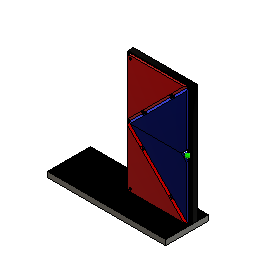
Evolution_door (Autodesk Fusion 360 design; units mm, degrees)
Autodesk Fusion 360 part; units mm, degrees
sketch "Frame" plane through (0, 0, 0) normal (0, 0, 1) x (1, 0, 0) in component "Door frame"
  line L0 (0, 0) -> (50, 0)
  line L1 (50, 0) -> (50, 100)
  line L2 (50, 100) -> (0, 100)
  line L3 (0, 100) -> (0, 0)
  line L4 (-5, -5) -> (55, -5)
  line L5 (55, -5) -> (55, 105)
  line L6 (55, 105) -> (-5, 105)
  line L7 (-5, 105) -> (-5, -5)
  dimension "d1" = 5
  constraint horizontal L0
  constraint vertical L1
  constraint horizontal L2
  constraint vertical L3
  constraint coincident L0.start L3.end
extrude "Extrude1" add sketch "Frame" against normal blind 5 makes body 1 in component "Door frame"
sketch "Body" plane through (0, 0, 0) normal (0, 0, 1) x (1, 0, 0) in component "Triangle1"
  line L0 (0, 0) -> (0, 100) construction
  line L1 (0, 100) -> (50, 100) construction
  line L2 (50, 100) -> (50, 0)
  line L3 (50, 0) -> (0, 0)
  line L4 (-5, 105) -> (-5, -5)
  line L5 (-5, -5) -> (55, -5)
  line L6 (55, -5) -> (55, 105)
  line L7 (55, 105) -> (-5, 105)
  line L8 (0, 100) -> (-5, 105) construction
  line L9 (50, 100) -> (55, 105) construction
  line L10 (-5, 50) -> (55, 50) construction
  line L11 (-2.5, 105) -> (-2.5, 50) construction
  line L12 (52.5, 105) -> (52.5, 50) construction
  line L13 (52.5, 105) -> (-2.5, 105) construction
  line L14 (52.5, 105) -> (-2.5, 50) construction
  line L15 (50, 100) -> (50, 105) construction
  line L16 (-2.5, 50) -> (-2.5, 52.5) construction
  line L17 (50, 105) -> (-2.5, 52.5)
  line L18 (-2.5, 52.5) -> (-2.5, 105)
  line L19 (-2.5, 105) -> (2.5, 105) construction
  line L20 (2.5, 105) -> (2.5, 100) construction
  line L21 (2.5, 100) -> (-2.5, 100) construction
  line L22 (-2.5, 100) -> (-2.5, 105) construction
  circle A0 centre (0, 102.5) radius 1.1
  line L23 (23.75, 78.75) -> (50, 105)
  line L24 (36.875, 91.875) -> (38.125, 90.625)
  line L25 (23.75, 78.75) -> (-2.5, 52.5)
  line L26 (10.625, 65.625) -> (11.875, 64.375)
  line L27 (10.625, 65.625) -> (11.3321, 66.3321)
  line L28 (11.3321, 66.3321) -> (12.5821, 65.0821)
  line L29 (11.875, 64.375) -> (12.5821, 65.0821)
  line L30 (36.875, 91.875) -> (37.5821, 92.5821)
  line L31 (37.5821, 92.5821) -> (38.8321, 91.3321)
  line L32 (38.125, 90.625) -> (38.8321, 91.3321)
  line L33 (11.875, 64.375) -> (12.5821, 63.6679)
  line L34 (12.5821, 65.0821) -> (13.2892, 64.375)
  line L35 (12.5821, 63.6679) -> (13.2892, 64.375)
  line L36 (11.875, 64.375) -> (11.1679, 65.0821)
  line L37 (11.1679, 65.0821) -> (11.875, 65.7892)
  line L38 (11.5214, 64.7286) -> (12.2286, 65.4357)
  line L39 (12.2286, 64.0214) -> (12.9357, 64.7286)
  line L40 (38.125, 90.625) -> (37.4179, 91.3321)
  line L41 (37.4179, 91.3321) -> (38.125, 92.0392)
  line L42 (37.7714, 90.9786) -> (38.4786, 91.6857)
  line L43 (38.125, 90.625) -> (38.8321, 89.9179)
  line L44 (38.8321, 91.3321) -> (39.5392, 90.625)
  line L45 (38.8321, 89.9179) -> (39.5392, 90.625)
  line L46 (38.4786, 90.2714) -> (39.1857, 90.9786)
  line L47 (-2.5, 52.5) -> (-2.5, 50.5)
  line L48 (10.625, 65.625) -> (9.2108, 64.2108)
  line L49 (36.875, 91.875) -> (35.4608, 90.4608)
  line L50 (-2.5, 50.5) -> (-2.5, 50)
  line L51 (10.8143, 63.3143) -> (-2.5, 50)
  line L52 (52.5, 105) -> (38.8321, 91.3321)
  line L53 (37.0643, 89.5643) -> (12.5821, 65.0821)
  line L54 (9.2108, 64.2108) -> (10.4608, 62.9608)
  line L55 (35.4608, 90.4608) -> (36.7101, 89.2101)
  line L56 (52.5, 105) -> (-2.5, 105)
  dimension "d4" = 2.5
  dimension "d5" = 5
  dimension "d6" = 5
  dimension "d7" = 2.2
  dimension "d43" = 1
  dimension "d44" = 1
  dimension "d45" = 1
  dimension "d46" = 1
  dimension "d47" = 1
  dimension "d48" = 1
  dimension "d49" = 1
  dimension "d50" = 1
  dimension "d196" = 2
  dimension "d198" = 2
  constraint coincident L0.end L1.start
  constraint coincident L4.start L7.end
  constraint coincident L1.end L2.start
  constraint coincident L6.end L7.start
  constraint midpoint L4 L10.start
  constraint midpoint L6 L10.end
  constraint coincident L7 L11.start
  constraint coincident L10 L11.end
  constraint perpendicular L10 L11
  constraint coincident L7 L12.start
  constraint coincident L13 L15.end
  constraint perpendicular L10 L16
  constraint horizontal L19
  constraint vertical L20
  constraint horizontal L21
  constraint vertical L22
  constraint midpoint L17 L23.start
  constraint midpoint L23 L24.start
  constraint coincident L14 L24.end
  constraint perpendicular L14 L24
  constraint midpoint L25 L26.start
  constraint coincident L14 L26.end
  constraint perpendicular L14 L26
  constraint perpendicular L26 L27
  constraint coincident L14 L28.end
  constraint perpendicular L14 L28
  constraint perpendicular L24 L30
  constraint coincident L14 L31.end
  constraint perpendicular L14 L31
  constraint perpendicular L29 L33
  constraint perpendicular L14 L34
  constraint perpendicular L29 L36
  constraint coincident L28 L37.end
  constraint perpendicular L28 L37
  constraint midpoint L36 L38.start
  constraint coincident L28 L38.end
  constraint perpendicular L28 L38
  constraint midpoint L33 L39.start
  constraint midpoint L34 L39.end
  constraint perpendicular L32 L40
  constraint coincident L31 L41.end
  constraint perpendicular L31 L41
  constraint midpoint L40 L42.start
  constraint perpendicular L24 L42
  constraint perpendicular L32 L43
  constraint perpendicular L32 L44
  constraint midpoint L43 L46.start
  constraint midpoint L44 L46.end
  constraint coincident L11 L47.end
  constraint parallel L11 L47
  constraint perpendicular L26 L48
  constraint perpendicular L24 L49
  constraint parallel L11 L50
  constraint coincident L14 L51.start
  constraint coincident L14 L53.start
  constraint coincident L51 L54.end
  constraint coincident L14 L54.end
  constraint coincident L53 L55.end
  measures "d4" distance of L11.end L16.end
  measures "d5" distance of L11.start L19.end
  measures "d6" distance of L11.start L21.end
  measures "d7" diameter of A0
  measures "d43" distance of L26.start L27.end
  measures "d44" distance of L24.start L30.end
  measures "d45" distance of L26.end L33.end
  measures "d46" distance of L28.end L34.end
  measures "d47" distance of L26.end L36.end
  measures "d48" distance of L24.end L40.end
  measures "d49" distance of L24.end L43.end
  measures "d50" distance of L31.end L44.end
  measures "d196" distance of L26.start L48.end
  measures "d198" distance of L24.start L49.end
extrude "Extrude1'" add sketch "Body" along normal blind 3 and the other way blind -1 separate body contours L7 L17 L18 L23 L25 L27 L30 L48 L49 L56 makes body 2 in component "Triangle1"
sketch "Triangle1 holder" plane through (0, 0, 0) normal (0, 0, 1) x (1, 0, 0) in component "Door frame"
  line L0 (0, 0) -> (0, 100)
  line L1 (0, 100) -> (50, 100)
  line L2 (50, 100) -> (50, 0)
  line L3 (50, 0) -> (0, 0)
  line L4 (-5, 105) -> (-5, -5)
  line L5 (-5, -5) -> (55, -5)
  line L6 (55, -5) -> (55, 105)
  line L7 (55, 105) -> (-5, 105)
  circle A0 centre (0, 102.5) radius 1
  circle A1 centre (0, 102.5) radius 1.5
  dimension "d12" = 2
  dimension "d13" = 3
  constraint concentric A0 A1
  measures "d12" diameter of A0
  measures "d13" diameter of A1
extrude "Extrude2" add sketch "Triangle1 holder" along normal blind 0.8 contours A1 bodies 1 in component "Door frame"
extrude "Extrude3" add 1 faces at (0.2444, 102.8261, 0) along direction (0, 0, 1) blind 3 on bodies 1 bodies 1 in component "Door frame"
sketch "Body (2)" plane through (0, 0, 0) normal (0, 0, 1) x (1, 0, 0) in component "Triangle4"
  line L0 (-5, 105) -> (-5, -5)
  line L1 (-5, -5) -> (55, -5)
  line L2 (55, -5) -> (55, 105)
  line L3 (55, 105) -> (-5, 105)
  line L4 (0, 0) -> (0, 100) construction
  line L5 (0, 100) -> (50, 100)
  line L6 (50, 100) -> (50, 0)
  line L7 (50, 0) -> (0, 0) construction
  circle A0 centre (0, 102.5) radius 1.5
  line L8 (-5, -5) -> (0, 0) construction
  line L9 (50, 0) -> (55, -5) construction
  line L10 (-5, 50) -> (55, 50) construction
  line L11 (52.5, -2.5) -> (52.5, -5) construction
  line L12 (-2.5, -2.5) -> (-2.5, -5) construction
  line L13 (-2.5, -5) -> (-2.5, 50) construction
  line L14 (52.5, -5) -> (52.5, 50) construction
  line L15 (50, 0) -> (50, -5) construction
  line L16 (-2.5, -5) -> (50, -5) construction
  line L17 (-2.5, -5) -> (-2.5, 47.5)
  line L18 (-2.5, 47.5) -> (50, -5)
  circle A1 centre (0, -2.5) radius 1.1
  line L19 (-2.5, 50) -> (52.5, -5) construction
  line L20 (23.75, 21.25) -> (50, -5)
  line L21 (36.875, 8.125) -> (38.125, 9.375)
  line L22 (-2.5, 47.5) -> (23.75, 21.25)
  line L23 (10.625, 34.375) -> (11.875, 35.625)
  line L24 (10.625, 34.375) -> (11.3321, 33.6679)
  line L25 (11.3321, 33.6679) -> (12.5821, 34.9179)
  line L26 (11.875, 35.625) -> (12.5821, 34.9179)
  line L27 (11.875, 35.625) -> (11.5214, 35.2714)
  line L28 (11.5214, 35.2714) -> (12.2286, 34.5643)
  line L29 (11.875, 35.625) -> (12.5821, 36.3321)
  line L30 (12.5821, 34.9179) -> (13.2892, 35.625)
  line L31 (12.5821, 36.3321) -> (13.2892, 35.625)
  line L32 (12.2286, 35.9786) -> (12.9357, 35.2714)
  line L33 (36.875, 8.125) -> (37.5821, 7.4179)
  line L34 (37.5821, 7.4179) -> (38.8321, 8.6679)
  line L35 (38.125, 9.375) -> (37.7714, 9.0214)
  line L36 (37.7714, 9.0214) -> (38.4786, 8.3143)
  line L37 (38.125, 9.375) -> (38.8321, 10.0821)
  line L38 (38.8321, 10.0821) -> (39.5392, 9.375)
  line L39 (39.5392, 9.375) -> (38.8321, 8.6679)
  line L40 (38.4786, 9.7286) -> (39.1857, 9.0214)
  line L41 (-2.5, 47.5) -> (-2.5, 50)
  line L42 (10.625, 34.375) -> (9.2108, 35.7892)
  line L43 (9.2108, 35.7892) -> (10.4608, 37.0392)
  line L44 (36.875, 8.125) -> (35.4608, 9.5392)
  line L45 (35.4608, 9.5392) -> (36.7108, 10.7892)
  line L46 (-2.5, 50) -> (10.4608, 37.0392)
  line L47 (12.5821, 34.9179) -> (36.7108, 10.7892)
  line L48 (38.8321, 8.6679) -> (52.5, -5)
  dimension "d25" = 2.2
  dimension "d61" = 1
  dimension "d62" = 0.5
  dimension "d63" = 1
  dimension "d64" = 1
  dimension "d65" = 1
  dimension "d66" = 0.5
  dimension "d67" = 1
  dimension "d206" = 2
  dimension "d207" = 2
  constraint coincident L0.end L1.start
  constraint coincident L4.start L7.end
  constraint coincident L6.end L7.start
  constraint coincident L1.end L2.start
  constraint midpoint L0 L10.start
  constraint perpendicular L0 L10
  constraint midpoint L9 L11.start
  constraint coincident L1 L11.end
  constraint perpendicular L1 L11
  constraint midpoint L8 L12.start
  constraint coincident L1 L12.end
  constraint perpendicular L1 L12
  constraint coincident L10 L13.end
  constraint perpendicular L10 L13
  constraint perpendicular L1 L14
  constraint coincident L13 L17.end
  constraint midpoint L18 L20.start
  constraint midpoint L20 L21.start
  constraint coincident L19 L21.end
  constraint perpendicular L19 L21
  constraint midpoint L22 L23.start
  constraint coincident L19 L23.end
  constraint perpendicular L19 L23
  constraint perpendicular L23 L24
  constraint coincident L19 L25.end
  constraint perpendicular L19 L25
  constraint perpendicular L26 L27
  constraint coincident L25 L28.end
  constraint perpendicular L25 L28
  constraint perpendicular L19 L29
  constraint perpendicular L19 L30
  constraint midpoint L29 L32.start
  constraint midpoint L30 L32.end
  constraint perpendicular L21 L33
  constraint coincident L19 L34.end
  constraint perpendicular L19 L34
  constraint perpendicular L19 L35
  constraint coincident L34 L36.end
  constraint perpendicular L34 L36
  constraint perpendicular L19 L37
  constraint perpendicular L37 L38
  constraint midpoint L37 L40.start
  constraint midpoint L39 L40.end
  constraint perpendicular L23 L42
  constraint coincident L19 L43.end
  constraint perpendicular L19 L43
  constraint perpendicular L43 L44
  constraint coincident L19 L45.end
  constraint perpendicular L19 L45
  measures "d25" diameter of A1
  measures "d61" distance of L23.start L24.end
  measures "d62" distance of L23.end L27.end
  measures "d63" distance of L23.end L29.end
  measures "d64" distance of L25.end L30.end
  measures "d65" distance of L21.start L33.end
  measures "d66" distance of L21.end L35.end
  measures "d67" distance of L21.end L37.end
  measures "d206" distance of L23.start L42.end
  measures "d207" distance of L21.start L44.end
extrude "Extrude1''" add sketch "Body (2)" along normal blind 3 and the other way blind -1 separate body contours L1 L17 L18 L20 L22 L24 L33 L42 L44 makes body 3 in component "Triangle4"
sketch "Sketch3" plane through (0, 0, 0) normal (0, 0, 1) x (1, 0, 0) in component "Door frame"
  line L0 (-5, 105) -> (-5, -5)
  line L1 (-5, -5) -> (55, -5)
  line L2 (55, -5) -> (55, 105)
  line L3 (55, 105) -> (-5, 105)
  line L4 (0, 0) -> (0, 100)
  line L5 (0, 100) -> (50, 100)
  line L6 (50, 100) -> (50, 0)
  line L7 (50, 0) -> (0, 0)
  circle A0 centre (0, 102.5) radius 1.5
  circle A1 centre (0, -2.5) radius 1
  circle A2 centre (0, -2.5) radius 1.5
  dimension "d30" = 2
  dimension "d31" = 3
  constraint concentric A1 A2
  measures "d30" diameter of A1
  measures "d31" diameter of A2
extrude "Extrude4" add sketch "Sketch3" along normal blind 0.8 contours A2 bodies 1 in component "Door frame"
extrude "Extrude5" add 1 faces at (0.5696, -2.7503, 0) along direction (0, 0, 1) blind 3 on bodies 1 bodies 1 in component "Door frame"
extrude "Extrude2'" add sketch "Body" along normal blind 3 and the other way blind -1 contours L17 L23 L24 L30 L31 L41 | L24 L31 L32 L40 L42 | L32 L43 L44 L46 | L24 L31 L40 L41 L42 | L17 L25 L26 L27 L28 L37 | L43 L44 L45 L46 | L26 L28 L36 L37 L38 | L26 L28 L29 L36 L38 | L29 L33 L34 L39 | L33 L34 L35 L39 bodies 2 in component "Triangle1"
extrude "Extrude3'" cut sketch "Body" along normal blind 2.5 and the other way blind -1.5 contours L24 L31 L32 L40 L42 | L32 L43 L44 L46 | L26 L28 L29 L36 L38 | L29 L33 L34 L39 bodies 2 in component "Triangle1"
fillet "Fillet2" radius 1 4 edges at (12.9357, 64.0214, 1) (12.9357, 64.0214, 3) (39.1857, 90.2714, 1) (39.1857, 90.2714, 3) on bodies 2 in component "Triangle1"
extrude "Extrude2''" add sketch "Body (2)" along normal blind 3 and the other way blind -1 contours L18 L20 L21 L33 L34 L36 | L21 L34 L35 L36 L37 L39 L40 | L18 L22 L23 L24 L25 L28 | L37 L38 L39 L40 | L23 L25 L26 L27 L28 | L26 L29 L30 L32 | L29 L30 L31 L32 bodies 3 in component "Triangle4"
extrude "Extrude3''" cut sketch "Body (2)" along normal blind 2.5 and the other way blind -1.5 contours L21 L34 L35 L36 L37 L39 L40 | L23 L25 L26 L27 L28 | L26 L29 L30 L32 bodies 3 in component "Triangle4"
fillet "Fillet1" radius 1 4 edges at (12.9357, 35.9786, 3) (12.9357, 35.9786, 1) (39.1857, 9.7286, 3) (39.1857, 9.7286, 1) on bodies 3 in component "Triangle4"
sketch "Body (3)" plane through (0, 0, 0) normal (0, 0, 1) x (1, 0, 0) in component "Triangle2"
  circle A0 centre (0, 102.5) radius 1.5
  line L0 (0, 0) -> (0, 100)
  line L1 (0, 100) -> (50, 100) construction
  line L2 (50, 100) -> (50, 0) construction
  line L3 (50, 0) -> (0, 0)
  line L4 (-5, 105) -> (-5, -5)
  line L5 (-5, -5) -> (55, -5)
  line L6 (55, -5) -> (55, 105)
  line L7 (55, 105) -> (-5, 105)
  circle A1 centre (0, -2.5) radius 1.5
  line L8 (-5, 105) -> (0, 100) construction
  line L9 (50, 100) -> (55, 105) construction
  line L10 (52.5, 102.5) -> (52.5, 105) construction
  line L11 (-2.5, 105) -> (-2.5, 50) construction
  line L12 (52.5, 105) -> (52.5, 50.7071) construction
  line L13 (-2.5, 50) -> (-2.5, 105) construction
  line L14 (-2.5, 50) -> (52.5, 105) construction
  line L15 (0, 50) -> (0, 52.5) construction
  line L16 (0, 50) -> (52.5, 102.5) construction
  line L17 (0, 52.5) -> (2.5, 52.5) construction
  line L18 (50, 100) -> (50, 102.5) construction
  line L19 (50, 100) -> (2.5, 52.5)
  line L20 (2.5, 52.5) -> (50, 52.5)
  line L21 (50, 52.5) -> (50, 100)
  line L22 (26.25, 76.25) -> (0, 50) construction
  line L23 (13.125, 63.125) -> (11.875, 64.375)
  line L24 (13.125, 63.125) -> (12.4179, 62.4179)
  line L25 (12.4179, 62.4179) -> (11.1679, 63.6679)
  line L26 (11.1679, 63.6679) -> (10.8143, 64.0214)
  line L27 (11.875, 64.375) -> (11.5214, 64.7286)
  line L28 (11.5214, 64.7286) -> (12.2293, 65.4364)
  line L29 (12.2293, 65.4364) -> (12.9371, 64.7286)
  line L30 (12.9371, 64.7286) -> (12.2293, 64.0207)
  line L31 (26.25, 76.25) -> (52.5, 102.5) construction
  line L32 (39.375, 89.375) -> (38.125, 90.625)
  line L33 (39.375, 89.375) -> (38.6679, 88.6679)
  line L34 (38.6679, 88.6679) -> (37.4179, 89.9179)
  line L35 (37.4179, 89.9179) -> (37.0643, 90.2714)
  line L36 (37.7714, 90.9786) -> (38.125, 90.625)
  line L37 (37.7714, 90.9786) -> (38.4786, 91.6857)
  line L38 (38.4786, 91.6857) -> (39.1857, 90.9786)
  line L39 (39.1857, 90.9786) -> (38.4786, 90.2714)
  line L40 (37.0643, 90.2714) -> (36.7108, 90.625)
  line L41 (37.7714, 90.9786) -> (37.4179, 91.3321)
  line L42 (36.7108, 90.625) -> (37.4179, 91.3321)
  line L43 (10.8143, 64.0214) -> (10.4608, 64.375)
  line L44 (11.5214, 64.7286) -> (11.1679, 65.0821)
  line L45 (11.1679, 65.0821) -> (10.4608, 64.375)
  line L46 (50, 52.5) -> (52.5, 50) construction
  line L47 (13.125, 63.125) -> (14.5392, 64.5392)
  line L48 (14.5392, 64.5392) -> (13.2892, 65.7892)
  line L49 (39.375, 89.375) -> (40.7892, 90.7892)
  line L50 (40.7892, 90.7892) -> (39.5392, 92.0392)
  line L51 (50, 102.5) -> (39.5392, 92.0392)
  line L52 (37.4179, 89.9179) -> (13.2892, 65.7892)
  line L53 (-2.5, 50) -> (11.1679, 63.6679)
  line L54 (50, 102.5) -> (52.5, 105)
  line L55 (52.5, 105) -> (52.5, 50.7071)
  line L56 (2.5, 52.5) -> (0, 50)
  line L57 (50, 100) -> (52.5, 102.5)
  line L58 (50, 52.5) -> (52.5, 55)
  line L59 (50, 52.5) -> (53.5355, 52.5) construction
  line L60 (50, 52.5) -> (47.5, 50)
  line L61 (50.3536, 52.8536) -> (52.8539, 50.3532)
  line L62 (52.8539, 50.3532) -> (52.1468, 49.6461)
  line L63 (52.1468, 49.6461) -> (49.6464, 52.1464)
  line L64 (51.7929, 50) -> (50, 50)
  line L65 (47.5, 50) -> (-2.5, 50)
  line L66 (50, 50) -> (47.5, 50)
  line L67 (52.5, 50.7071) -> (52.5, 50) construction
  line L68 (-5, 50) -> (51.7929, 50) construction
  line L69 (52.5, 50) -> (55, 50) construction
  line L70 (51.7929, 50) -> (52.5, 50) construction
  line L71 (52.5, 50) -> (51.7929, 50) construction
  line L72 (52.5, 50.7071) -> (52.5, 50) construction
  dimension "d77" = 1
  dimension "d78" = 0.5
  dimension "d79" = 0.5
  dimension "d80" = 1
  dimension "d81" = 0.5
  dimension "d82" = 1
  dimension "d83" = 1
  dimension "d84" = 1
  dimension "d94" = 0.5
  dimension "d95" = 0.5
  dimension "d96" = 0.5
  dimension "d97" = 0.5
  dimension "d214" = 2
  dimension "d215" = 2
  dimension "d252" = 45
  dimension "d254" = 3.536
  dimension "d255" = 1
  constraint midpoint L4 L68.start
  constraint midpoint L6 L69.end
  constraint coincident L4.start L7.end
  constraint coincident L0.end L1.start
  constraint coincident L1.end L2.start
  constraint coincident L6.end L7.start
  constraint midpoint L9 L10.start
  constraint coincident L7 L10.end
  constraint perpendicular L7 L10
  constraint coincident L7 L11.start
  constraint coincident L11.end L68
  constraint perpendicular L11 L68
  constraint coincident L46.end L68
  constraint perpendicular L12 L68
  constraint midpoint L0 L15.start
  constraint coincident L0 L15.end
  constraint coincident L14 L15.end
  constraint coincident L16 L17.end
  constraint perpendicular L15 L17
  constraint coincident L14 L18.end
  constraint perpendicular L1 L18
  constraint coincident L2 L20.end
  constraint perpendicular L2 L20
  constraint midpoint L19 L22.start
  constraint midpoint L22 L23.start
  constraint coincident L14 L23.end
  constraint perpendicular L14 L23
  constraint perpendicular L23 L24
  constraint coincident L14 L25.end
  constraint perpendicular L14 L25
  constraint perpendicular L14 L26
  constraint perpendicular L14 L27
  constraint perpendicular L27 L28
  constraint perpendicular L28 L29
  constraint coincident L23 L30.end
  constraint perpendicular L23 L30
  constraint midpoint L31 L32.start
  constraint coincident L14 L32.end
  constraint perpendicular L14 L32
  constraint perpendicular L32 L33
  constraint coincident L14 L34.end
  constraint perpendicular L14 L34
  constraint perpendicular L14 L35
  constraint perpendicular L36 L37
  constraint perpendicular L37 L38
  constraint coincident L32 L39.end
  constraint perpendicular L32 L39
  constraint parallel L35 L40
  constraint perpendicular L37 L41
  constraint perpendicular L41 L42
  constraint parallel L26 L43
  constraint perpendicular L28 L44
  constraint perpendicular L23 L47
  constraint coincident L14 L48.end
  constraint perpendicular L14 L48
  constraint perpendicular L32 L49
  constraint coincident L14 L50.end
  constraint perpendicular L14 L50
  constraint coincident L15.end L53
  constraint horizontal L59
  constraint coincident L55 L58.end
  constraint coincident L60.end L64
  constraint parallel L58 L60
  constraint perpendicular L46 L62
  constraint coincident L60 L63.end
  constraint perpendicular L60 L63
  constraint coincident L2 L64.end
  constraint coincident L61 L12.end
  constraint perpendicular L67 L68
  constraint coincident L63 L64.start
  constraint coincident L60.end L71
  constraint coincident L58.end L72
  measures "d77" distance of L23.start L24.end
  measures "d78" distance of L25.end L26.end
  measures "d79" distance of L23.end L27.end
  measures "d80" distance of L32.start L33.end
  measures "d81" distance of L34.end L35.end
  measures "d82" distance of L35.end L36.start
  measures "d83" distance of L36.start L37.end
  measures "d84" distance of L37.end L38.end
  measures "d94" distance of L35.end L40.end
  measures "d95" distance of L36.start L41.end
  measures "d96" distance of L26.end L43.end
  measures "d97" distance of L27.end L44.end
  measures "d214" distance of L23.start L47.end
  measures "d215" distance of L32.start L49.end
  measures "d252" angle of L58 L59
  measures "d254" distance of L61.start L61.end
  measures "d255" distance of L61.end L62.end
extrude "Extrude1'''" add sketch "Body (3)" along normal blind 3 and the other way blind -1 separate body contours L20 L56 L60 L65 | L19 L20 L21 L24 L33 L47 L49 | L19 L23 L24 L25 L26 L27 L43 L44 L45 | L21 L55 L57 L58 | L19 L32 L33 L34 L35 L36 L40 L41 L42 makes body 4 in component "Triangle2"
extrude "Extrude2'''" add sketch "Body (3)" along normal blind 2.5 and the other way blind -1.5 contours L23 L27 L28 L29 L30 | L32 L36 L37 L38 L39 bodies 4 in component "Triangle2"
fillet "Fillet1'" radius 0.5 8 edges at (11.8754, 65.0825, 2.5) (12.5832, 64.3746, 2.5) (11.8754, 65.0825, 1.5) (12.5832, 64.3746, 1.5) (38.125, 91.3321, 1.5) (38.8321, 90.625, 1.5) (38.125, 91.3321, 2.5) (38.8321, 90.625, 2.5) on bodies 4 in component "Triangle2"
fillet "Fillet2'" radius 1 4 edges at (37.0643, 90.9786, 3) (37.0643, 90.9786, 1) (10.8143, 64.7286, 1) (10.8143, 64.7286, 3) on bodies 4 in component "Triangle2"
sketch "Body (4)" plane through (0, 0, 0) normal (0, 0, 1) x (1, 0, 0) in component "Triangle3"
  circle A0 centre (0, 102.5) radius 1.5
  line L0 (0, 0) -> (0, 100) construction
  line L1 (0, 100) -> (50, 100)
  line L2 (50, 100) -> (50, 0) construction
  line L3 (50, 0) -> (0, 0) construction
  line L4 (-5, 105) -> (-5, -5)
  line L5 (-5, -5) -> (55, -5)
  line L6 (55, -5) -> (55, 105)
  line L7 (55, 105) -> (-5, 105)
  circle A1 centre (0, -2.5) radius 1.5
  line L8 (-5, 50) -> (55, 50) construction
  line L9 (-5, -5) -> (0, 0) construction
  line L10 (55, -5) -> (50, 0) construction
  line L11 (52.5, -2.5) -> (52.5, -5) construction
  line L12 (-2.5, -2.5) -> (-2.5, -5) construction
  line L13 (-2.5, -5) -> (-2.5, 50) construction
  line L14 (52.5, -5) -> (52.5, 50) construction
  line L15 (-2.5, 50) -> (52.5, -5) construction
  line L16 (-2.5, 50) -> (0, 50) construction
  line L17 (0, 47.5) -> (2.5, 47.5) construction
  line L18 (50, 0) -> (50, -2.5) construction
  line L19 (2.5, 47.5) -> (50, 0)
  line L20 (2.5, 47.5) -> (50, 47.5)
  line L21 (50, 47.5) -> (50, 0)
  line L22 (0, 50) -> (52.5, -2.5) construction
  line L23 (26.25, 23.75) -> (0, 50) construction
  line L24 (13.125, 36.875) -> (11.875, 35.625)
  line L25 (11.875, 35.625) -> (11.1679, 34.9179)
  line L26 (13.125, 36.875) -> (12.4179, 37.5821)
  line L27 (12.4179, 37.5821) -> (11.1679, 36.3321)
  line L28 (11.1679, 36.3321) -> (10.4608, 35.625)
  line L29 (11.1679, 34.9179) -> (10.4608, 35.625)
  line L30 (11.5214, 35.2714) -> (10.8143, 35.9786)
  line L31 (11.875, 35.625) -> (12.2286, 35.9786)
  line L32 (12.2286, 35.9786) -> (11.5214, 36.6857)
  line L33 (26.25, 23.75) -> (52.5, -2.5) construction
  line L34 (39.375, 10.625) -> (38.125, 9.375)
  line L35 (39.375, 10.625) -> (38.6679, 11.3321)
  line L36 (38.6679, 11.3321) -> (37.4179, 10.0821)
  line L37 (37.4179, 10.0821) -> (36.7108, 9.375)
  line L38 (38.125, 9.375) -> (37.4179, 8.6679)
  line L39 (37.4179, 8.6679) -> (36.7108, 9.375)
  line L40 (37.7714, 9.0214) -> (37.0643, 9.7286)
  line L41 (38.125, 9.375) -> (38.4786, 9.7286)
  line L42 (38.4786, 9.7286) -> (37.7714, 10.4357)
  line L43 (11.5214, 35.2714) -> (12.2286, 34.5643)
  line L44 (12.2286, 34.5643) -> (12.9357, 35.2714)
  line L45 (12.9357, 35.2714) -> (12.2286, 35.9786)
  line L46 (37.7714, 9.0214) -> (38.4786, 8.3143)
  line L47 (38.4786, 8.3143) -> (39.1857, 9.0214)
  line L48 (39.1857, 9.0214) -> (38.4786, 9.7286)
  line L49 (50, 47.5) -> (52.5, 50) construction
  line L50 (51.25, 48.75) -> (51.6036, 48.3964) construction
  line L51 (13.125, 36.875) -> (14.5392, 35.4608)
  line L52 (14.5392, 35.4608) -> (13.2892, 34.2108)
  line L53 (13.2892, 34.2108) -> (37.4179, 10.0821)
  line L54 (39.375, 10.625) -> (40.7892, 9.2108)
  line L55 (40.7892, 9.2108) -> (39.5392, 7.9608)
  line L56 (39.5392, 7.9608) -> (52.5, -5)
  line L57 (11.1679, 36.3321) -> (-2.5, 50)
  line L58 (-2.5, 50) -> (51.7929, 50)
  line L59 (52.5, 49.2929) -> (52.5, -5)
  line L60 (50, 0) -> (52.5, -2.5)
  line L61 (2.5, 47.5) -> (0, 50)
  line L62 (50, 47.5) -> (52.5, 45)
  line L63 (50, 47.5) -> (47.5, 50)
  line L64 (50.3536, 47.1464) -> (52.8539, 49.6468)
  line L65 (52.8539, 49.6468) -> (52.1468, 50.3539)
  line L66 (52.1468, 50.3539) -> (49.6464, 47.8536)
  dimension "d106" = 1
  dimension "d107" = 1
  dimension "d108" = 1
  dimension "d109" = 0.5
  dimension "d110" = 1
  dimension "d111" = 1
  dimension "d112" = 1
  dimension "d113" = 0.5
  dimension "d118" = 1
  dimension "d119" = 1
  dimension "d120" = 1
  dimension "d121" = 1
  dimension "d147" = 0.5
  dimension "d222" = 2
  dimension "d223" = 2
  dimension "d256" = 0.5
  dimension "d257" = 3.536
  dimension "d258" = 1
  constraint midpoint L4 L8.start
  constraint midpoint L6 L8.end
  constraint coincident L4.end L5.start
  constraint coincident L0.start L3.end
  constraint coincident L5.end L6.start
  constraint coincident L2.end L3.start
  constraint midpoint L10 L11.start
  constraint coincident L5 L11.end
  constraint perpendicular L5 L11
  constraint midpoint L9 L12.start
  constraint coincident L5 L12.end
  constraint perpendicular L5 L12
  constraint parallel L0 L13
  constraint perpendicular L5 L14
  constraint midpoint L0 L16.end
  constraint perpendicular L0 L16
  constraint coincident L0 L17.start
  constraint coincident L15 L17.start
  constraint perpendicular L0 L17
  constraint coincident L15 L18.end
  constraint perpendicular L3 L18
  constraint coincident L2 L20.end
  constraint perpendicular L2 L20
  constraint midpoint L22 L23.start
  constraint midpoint L23 L24.start
  constraint coincident L15 L24.end
  constraint perpendicular L15 L24
  constraint perpendicular L15 L25
  constraint perpendicular L24 L26
  constraint coincident L15 L27.end
  constraint perpendicular L15 L27
  constraint perpendicular L15 L28
  constraint midpoint L25 L30.start
  constraint midpoint L28 L30.end
  constraint perpendicular L15 L31
  constraint coincident L27 L32.end
  constraint perpendicular L27 L32
  constraint midpoint L33 L34.start
  constraint coincident L15 L34.end
  constraint perpendicular L15 L34
  constraint perpendicular L34 L35
  constraint coincident L15 L36.end
  constraint perpendicular L15 L36
  constraint perpendicular L15 L37
  constraint perpendicular L15 L38
  constraint midpoint L38 L40.start
  constraint midpoint L37 L40.end
  constraint perpendicular L15 L41
  constraint coincident L36 L42.end
  constraint perpendicular L36 L42
  constraint perpendicular L25 L43
  constraint perpendicular L43 L44
  constraint perpendicular L38 L46
  constraint perpendicular L46 L47
  constraint midpoint L49 L50.start
  constraint perpendicular L49 L50
  constraint perpendicular L24 L51
  constraint coincident L15 L52.end
  constraint perpendicular L15 L52
  constraint perpendicular L34 L54
  constraint coincident L15 L55.end
  constraint perpendicular L15 L55
  constraint parallel L22 L61
  constraint coincident L14 L62.end
  constraint perpendicular L49 L62
  constraint coincident L8 L63.end
  constraint coincident L58 L63.end
  constraint perpendicular L49 L65
  constraint coincident L63 L66.end
  constraint perpendicular L63 L66
  constraint coincident L66 L58.end
  constraint coincident L64 L59.start
  measures "d106" distance of L24.end L25.end
  measures "d107" distance of L24.start L26.end
  measures "d108" distance of L27.end L28.end
  measures "d109" distance of L24.end L31.end
  measures "d110" distance of L34.start L35.end
  measures "d111" distance of L36.end L37.end
  measures "d112" distance of L34.end L38.end
  measures "d113" distance of L34.end L41.end
  measures "d118" distance of L30.start L43.end
  measures "d119" distance of L43.end L44.end
  measures "d120" distance of L40.start L46.end
  measures "d121" distance of L46.end L47.end
  measures "d147" distance of L50.start L50.end
  measures "d222" distance of L24.start L51.end
  measures "d223" distance of L34.start L54.end
  measures "d256" distance of L20.end L64.start
  measures "d257" distance of L64.start L64.end
  measures "d258" distance of L64.end L65.end
extrude "Extrude1''''" add sketch "Body (4)" along normal blind 3 and the other way blind -1 separate body contours L21 L59 L60 L62 | L19 L20 L21 L26 L35 L51 L54 | L19 L34 L35 L36 L42 | L20 L58 L61 L63 | L34 L36 L37 L38 L40 L41 L42 | L19 L24 L26 L27 L32 | L37 L38 L39 L40 | L24 L25 L27 L28 L30 L31 L32 | L25 L28 L29 L30 makes body 5 in component "Triangle3"
extrude "Extrude2''''" add sketch "Body (4)" along normal blind 2.5 and the other way blind -1.5 contours L34 L38 L41 L46 L47 L48 | L24 L25 L31 L43 L44 L45 bodies 5 in component "Triangle3"
fillet "Fillet1''" radius 0.5 8 edges at (12.5821, 35.625, 2.5) (11.875, 34.9179, 2.5) (12.5821, 35.625, 1.5) (11.875, 34.9179, 1.5) (38.125, 8.6679, 1.5) (38.8321, 9.375, 1.5) (38.8321, 9.375, 2.5) (38.125, 8.6679, 2.5) on bodies 5 in component "Triangle3"
fillet "Fillet2''" radius 1 4 edges at (37.0643, 9.0214, 1) (37.0643, 9.0214, 3) (10.8143, 35.2714, 3) (10.8143, 35.2714, 1) on bodies 5 in component "Triangle3"
ref_plane "WorkPlane1" through (52.5, 21.25, 2) normal (1, 0, 0) x (0, 1, 0)
extrude "Extrude4'" add sketch "Body (4)" along normal blind 3 and the other way blind -1 contours L19 L55 L56 L59 L60 | L19 L36 L52 L53 | L19 L27 L57 L58 L61 bodies 5 in component "Triangle3"
chamfer "Chamfer1" distance 1.767 distance2 2 3 edges at (4.3339, 43.1661, 3) (25.3536, 22.1464, 3) (46.0196, 1.4804, 3) measured on face at (34.6381, 31.1953, 3) measured on face at (34.6381, 31.1953, 3) measured on face at (34.6381, 31.1953, 3) on bodies 5 in component "Triangle3"
extrude "Extrude4''" add sketch "Body" along normal blind 3 and the other way blind -1 contours L7 L17 L23 L31 L52 L56 | L17 L25 L47 L50 L51 L54 | L17 L23 L25 L28 L53 L55 bodies 2 in component "Triangle1"
chamfer "Chamfer1'" distance 1.767 distance2 2 3 edges at (24.6461, 77.1461, 3) (45.6661, 98.1661, 3) (3.9804, 56.4804, 3) measured on face at (15.5905, 85.9086, 3) measured on face at (15.5905, 85.9086, 3) measured on face at (15.5905, 85.9086, 3) on bodies 2 in component "Triangle1"
extrude "Extrude4'''" add sketch "Body (2)" along normal blind 3 and the other way blind -1 contours L1 L18 L20 L34 L48 | L18 L22 L41 L43 L46 | L18 L20 L22 L25 L45 L47 bodies 3 in component "Triangle4"
chamfer "Chamfer1''" distance 1.768 distance2 2 3 edges at (45.6661, 1.8339, 3) (24.6464, 22.8536, 3) (3.9804, 43.5196, 3) measured on face at (15.5905, 14.0914, 3) measured on face at (15.5905, 14.0914, 3) measured on face at (15.5905, 14.0914, 3) on bodies 3 in component "Triangle4"
extrude "Extrude6" add sketch "Body (3)" along normal blind 3 and the other way blind -1 contours L0 L53 L65 | L0 L19 L25 L53 L56 | L19 L50 L51 L54 L55 L57 | L19 L34 L48 L52 bodies 4 in component "Triangle2"
chamfer "Chamfer1'''" distance 1.767 distance2 2 3 edges at (4.3339, 56.8339, 3) (25.3536, 77.8536, 3) (46.0196, 98.5196, 3) measured on face at (35.4714, 69.6381, 3) measured on face at (35.4714, 69.6381, 3) measured on face at (35.4714, 69.6381, 3) on bodies 4 in component "Triangle2"
sphere "SpherePrimitive2" add diameter 4 placed x (0, 0, -1) y (0, 1, 0) z (1, 0, 0) at (52.5, 50, 2) separate body makes body 6 in component "Kniob"
fillet "Fillet3" radius 2.5 1 edges at (-2.5, 105, 2) on bodies 2 in component "Triangle1"
fillet "Fillet2'''" radius 2.5 1 edges at (-2.5, -5, 2) on bodies 3 in component "Triangle4"
sketch "Knob arm" plane through (48.75, 48.75, 0) normal (0.707107, 0.707107, 0) x (0, 0, -1) in component "Triangle3"
  line L0 (-1, -1.7678) -> (-1, 1.7678)
  line L1 (-1, 1.7678) -> (-3, 1.7678)
  line L2 (-3, 1.7678) -> (-3, -1.7678)
  line L3 (-3, -1.7678) -> (-1, -1.7678)
  circle A0 centre (-2, -1.7678) radius 0.5
  dimension "d261" = 1
  constraint midpoint L3 A0.centre
  measures "d261" diameter of A0
extrude "Extrude5'" add sketch "Knob arm" along normal blind 3.536 contours L3 A0 | L3 A0 bodies 5 in component "Triangle3"
sketch "Knob arm (2)" plane through (-1.25, 1.25, 0) normal (0.707107, -0.707107, 0) x (0, 0, -1) in component "Triangle2"
  line L0 (-1, 68.9429) -> (-1, 76.014)
  line L1 (-1, 76.014) -> (-3, 76.014)
  line L2 (-3, 76.014) -> (-3, 68.9429)
  line L3 (-3, 68.9429) -> (-1, 68.9429)
  circle A0 centre (-2, 72.5) radius 0.5
  dimension "d264" = 1
  measures "d264" diameter of A0
extrude "Extrude8" add sketch "Knob arm (2)" along normal blind 3.536 contours A0 bodies 4 in component "Triangle2"
sketch "Sketch5" plane through (0, -5, 0) normal (0, -1, 0) x (1, 0, 0)
  line L0 (55, 0) -> (-5, 0)
  line L1 (-5, 0) -> (-5, -5)
  line L2 (-5, -5) -> (55, -5)
  line L3 (55, -5) -> (55, 0)
sketch "Holder" plane through (0, 0, 0) normal (0, 1, 0) x (1, 0, 0) in component "Holder"
  line L0 (55, 15) -> (-55, 15)
  line L1 (-55, 15) -> (-55, -25)
  line L2 (-55, -25) -> (55, -25)
  line L3 (55, -25) -> (55, 15)
  constraint horizontal L0
  constraint vertical L1
  constraint horizontal L2
  constraint vertical L3
extrude "Extrude1'''''" add sketch "Holder" along normal blind -10 and the other way blind 5 separate body makes body 7 in component "Holder"
chamfer "Chamfer2" [suppressed] in component "Triangle1"
chamfer "Chamfer2'" [no effect] in component "Triangle4"
component "Door frame" placed x (1, 0, 0) y (0, 1, 0) z (0, 0, 1) at (0, 0, 0)
component "Triangle1" placed x (1, 0, 0) y (0, 1, 0) z (0, 0, 1) at (0, 0, 0)
component "Triangle4" placed x (1, 0, 0) y (0, 1, 0) z (0, 0, 1) at (0, 0, 0)
component "Triangle2" placed x (1, 0, 0) y (0, 1, 0) z (0, 0, 1) at (0, 0, 0)
component "Triangle3" placed x (1, 0, 0) y (0, 1, 0) z (0, 0, 1) at (0, 0, 0)
component "Kniob" placed x (1, 0, 0) y (0, 1, 0) z (0, 0, 1) at (0, 0, 0)
component "Holder" placed x (1, 0, 0) y (0, 1, 0) z (0, 0, 1) at (0, 0, 0)
named bodies: "Frame", "Body", "Knob", "Holder"
